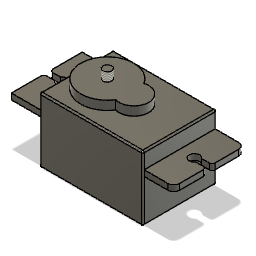
ServoMotor representação v3 (Autodesk Fusion 360 design; units mm, degrees)
Autodesk Fusion 360 part; units mm, degrees
sketch "Sketch1" plane through (0, 0, 0) normal (0, 1, 0) x (1, 0, 0)
  line L0 (0, 0) -> (35, 0)
  line L1 (35, 0) -> (35, -25)
  line L2 (35, -25) -> (0, -25)
  line L3 (0, -25) -> (0, 0)
  dimension "d1" = 35
  dimension "d2" = 25
  constraint horizontal L0
  constraint vertical L1
  constraint horizontal L2
  constraint vertical L3
  constraint coincident L0.start L3.end
  measures "d1" distance of L0.start L0.end
  measures "d2" distance of L0.start L2.end
extrude "Extrude1" add sketch "Sketch1" along normal blind 22 makes body 1
fillet "Fillet1" radius 0.5 12 edges at (35, 22, 12.5) (17.5, 22, 25) (0, 22, 12.5) (17.5, 22, 0) (17.5, 0, 25) (35, 0, 12.5) (35, 11, 0) (35, 11, 25) (17.5, 0, 0) (0, 11, 0) (0, 11, 25) (0, 0, 12.5) on bodies 1
sketch "Sketch2" plane through (0, 22, 0) normal (0, 1, 0) x (-1, 0, 0)
  line L0 (-34.5, 0.5) -> (-0.5, 0.5)
  line L1 (-0.5, 0.5) -> (-0.5, 24.5)
  line L2 (-0.5, 24.5) -> (-34.5, 24.5)
  line L3 (-34.5, 24.5) -> (-34.5, 0.5)
  arc A0 (-18.1111, 17.3032) -> (-18.1111, 7.6968) centre (-19.5, 12.5) ccw
  arc A1 (-18.1111, 7.6968) -> (-18.1111, 17.3032) centre (-10.5, 12.5) ccw
  dimension "d8" = 18
  measures "d8" diameter of A1
extrude "Extrude2" add sketch "Sketch2" along normal blind 3 contours A0 A1 bodies 1
sketch "Sketch3" plane through (0, 25, 0) normal (0, 1, 0) x (-1, 0, 0)
  arc A0 (-18.1111, 7.6968) -> (-18.1111, 17.3032) centre (-10.5, 12.5) ccw
  arc A1 (-18.1111, 17.3032) -> (-18.1111, 7.6968) centre (-19.5, 12.5) ccw
  circle A2 centre (-10.5, 12.5) radius 1.5
  dimension "d20" = 3
  constraint concentric A0 A2
  measures "d20" diameter of A2
extrude "Extrude3" add sketch "Sketch3" along normal blind 3 contours A2 bodies 1
thread "Thread1" "ISO Metric profile 3.0 M3x0.5 6g" major diameter 2.927 minor diameter 2.3555 pitch 0.5 angle 60 resizes the face on face at (9.0019, 27, 12.4252) on bodies 1
sketch "Sketch4" plane through (35, 0, 0) normal (1, 0, 0) x (0, 0, -1)
  line L0 (-24.5, 0.5) -> (-0.5, 0.5)
  line L1 (-0.5, 0.5) -> (-0.5, 21.5)
  line L2 (-0.5, 21.5) -> (-24.5, 21.5)
  line L3 (-24.5, 21.5) -> (-24.5, 0.5)
  line L4 (-12.5, 21.5) -> (-12.5, 16.5)
  line L5 (-12.5, 16.5) -> (-24.5, 16.5)
  line L6 (-12.5, 16.5) -> (-0.5, 16.5)
  line L7 (-24.5, 16.5) -> (-24.5, 14.5)
  line L8 (-24.5, 14.5) -> (-0.5, 14.5)
  line L9 (-0.5, 14.5) -> (-0.5, 16.5)
  dimension "d23" = 5
  dimension "d24" = 12
  dimension "d25" = 12
  dimension "d26" = 2
  dimension "d27" = 24
  constraint midpoint L2 L4.start
  constraint perpendicular L2 L4
  constraint perpendicular L3 L5
  constraint perpendicular L4 L6
  constraint perpendicular L5 L7
  constraint perpendicular L7 L8
  measures "d23" distance of L4.start L4.end
  measures "d24" distance of L4.end L5.end
  measures "d25" distance of L4.end L6.end
  measures "d26" distance of L5.end L7.end
  measures "d27" distance of L7.end L8.end
extrude "Extrude4" add sketch "Sketch4" along normal blind 10 contours L1 L3 L5 L6 L7 L8 L9 bodies 1
fillet "Fillet2" radius 2 2 edges at (45, 15.5, 24.5) (45, 15.5, 0.5) on bodies 1
sketch "Sketch5" plane through (0, 16.5, 0) normal (0, 1, 0) x (-1, 0, 0)
  arc A0 (-45, 2.5) -> (-43, 0.5) centre (-43, 2.5) ccw
  line L0 (-43, 0.5) -> (-35, 0.5)
  line L1 (-35, 0.5) -> (-35, 24.5)
  line L2 (-35, 24.5) -> (-43, 24.5)
  arc A1 (-43, 24.5) -> (-45, 22.5) centre (-43, 22.5) ccw
  line L3 (-45, 22.5) -> (-45, 2.5)
  line L4 (-45, 12.5) -> (-45, 11.5)
  line L5 (-45, 12.5) -> (-45, 13.5)
  line L6 (-45, 13.5) -> (-41.4361, 13.5)
  line L7 (-45, 11.5) -> (-41.4361, 11.5)
  arc A2 (-41.4361, 11.5) -> (-41.4361, 13.5) centre (-40, 12.5) ccw
  dimension "d32" = 5
  dimension "d33" = 3.5
  dimension "d34" = 1
  dimension "d35" = 1
  constraint midpoint L3 L4.start
  constraint coincident L3 L5.end
  constraint perpendicular L5 L6
  constraint perpendicular L3 L7
  measures "d32" distance of L4.start A2.centre
  measures "d33" diameter of A2
  measures "d34" distance of L4.start L4.end
  measures "d35" distance of L4.start L5.end
extrude "Extrude5" cut sketch "Sketch5" against normal blind 6.2 contours L3 L4 L5 L6 L7 A2 bodies 1
fillet "Fillet3" radius 1 2 edges at (45, 15.5, 11.5) (45, 15.5, 13.5) on bodies 1
sketch "Sketch6" plane through (0, 0, 0) normal (-1, 0, 0) x (0, 0, 1)
  line L0 (24.5, 0.5) -> (24.5, 21.5)
  line L1 (24.5, 21.5) -> (0.5, 21.5)
  line L2 (0.5, 21.5) -> (0.5, 0.5)
  line L3 (0.5, 0.5) -> (24.5, 0.5)
  line L4 (0.5, 16.5) -> (24.5, 16.5)
  line L5 (24.5, 16.5) -> (24.5, 14.5)
  line L6 (24.5, 14.5) -> (0.5, 14.5)
  line L7 (0.5, 14.5) -> (0.5, 16.5)
  dimension "d40" = 5
  dimension "d41" = 24
  dimension "d42" = 2
  constraint horizontal L4
  constraint vertical L5
  constraint horizontal L6
  constraint vertical L7
  measures "d40" distance of L1.end L4.start
  measures "d41" distance of L4.start L4.end
  measures "d42" distance of L4.start L6.end
extrude "Extrude6" add sketch "Sketch6" along normal blind 10 contours L0 L2 L4 L5 L6 L7 bodies 1
sketch "Sketch7" plane through (0, 16.5, 0) normal (0, 1, 0) x (-1, 0, 0)
  line L0 (0, 24.5) -> (0, 0.5)
  line L1 (0, 0.5) -> (10, 0.5)
  line L2 (10, 0.5) -> (10, 24.5)
  line L3 (10, 24.5) -> (0, 24.5)
  line L4 (0, 12.5) -> (5, 12.5)
  line L5 (10, 12.5) -> (10, 11.5)
  line L6 (10, 12.5) -> (10, 13.5)
  line L7 (10, 11.5) -> (6.4361, 11.5)
  line L8 (10, 13.5) -> (6.4361, 13.5)
  arc A0 (6.4361, 13.5) -> (6.4361, 11.5) centre (5, 12.5) ccw
  dimension "d45" = 5
  dimension "d46" = 3.5
  dimension "d47" = 1
  dimension "d48" = 1
  constraint midpoint L0 L4.start
  constraint perpendicular L0 L4
  constraint coincident L4.end A0.centre
  constraint midpoint L2 L5.start
  constraint perpendicular L5 L7
  constraint perpendicular L6 L8
  measures "d45" distance of L4.start L4.end
  measures "d46" diameter of A0
  measures "d47" distance of L5.start L5.end
  measures "d48" distance of L5.start L6.end
extrude "Extrude7" cut sketch "Sketch7" against normal blind 6.5 contours L2 L5 L6 L7 L8 A0 bodies 1
fillet "Fillet4" radius 1 2 edges at (-10, 15.5, 13.5) (-10, 15.5, 11.5) on bodies 1
copy_body "Body->Comp1" bodies 1 removing the originals makes body 2 in component "Component"
component "Component" placed x (1, 0, 0) y (0, 1, 0) z (0, 0, 1) at (0, 0, 0)
